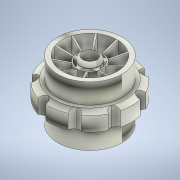
# Autodesk Inventor part: ozubene-kolo_mini
Saved by Autodesk Inventor 2022 (Build 260153000, 153)
## iProperties
Created: 2022-11-27
Part Number: ozubene-kolo_mini
Material: Generic
Document SubType Name: Modeling
Designer: matys
Density: 1 g/cm^3
Appearance: Running - Light Gray
Author: matys
Autodesk Inventor part; units mm, degrees
ref_plane "YZ Plane" through (0, 0, 0) normal (1, 0, 0) x (0, 1, 0)
ref_plane "XZ Plane" through (0, 0, 0) normal (0, 1, 0) x (-1, 0, 0)
ref_plane "XY Plane" through (0, 0, 0) normal (0, 0, 1) x (1, 0, 0)
sketch "Sketch1" plane through (0, 0, 0) normal (0, 1, 0) x (-1, 0, 0)
  line L0 (0, 0) -> (15, 0)
  circle A0 centre (0, 0) radius 15
  dimension "d0" = 15
  constraints: 2 end point, 1 coincident, 1 horizontal, 1 horizontal alignment, 2 other
  measures "d0" distance of L0.start L0.end
extrude "Extrusion1" add sketch "Sketch1" along normal blind 8.5
sketch "Sketch2" plane through (0, 8.5, 0) normal (0, 1, 0) x (1, 0, 0)
  line L0 (0, 0) -> (-15, 0)
  circle A0 centre (0, 0) radius 15 projected
  line L1 (-15, 0) -> (-19, 0)
  circle A1 centre (0, 0) radius 15
  line L2 (-15, 0) -> (-17.5, 0)
  circle A2 centre (0, 0) radius 17.5
  dimension "d10" = 2.5
  constraints: 6 end point, 2 coincident, 2 horizontal alignment, 2 point on line, 1 centre point, 1 horizontal, 4 other
  measures "d10" distance of L0.end L2.end
extrude "Extrusion2" add sketch "Sketch2" along normal blind 8 contours A0 | A2
sketch "Sketch3" plane through (0, 16.5, 0) normal (0, 1, 0) x (1, 0, 0)
  line L0 (0, 0) -> (-15, 0)
  circle A0 centre (0, 0) radius 15
  constraints: 2 end point, 1 coincident, 1 horizontal, 1 horizontal alignment, 2 other
extrude "Extrusion3" add sketch "Sketch3" along normal blind 8.5
sketch "Sketch5" plane through (0, 16.5, 0) normal (0, 1, 0) x (1, 0, 0)
  circle A0 centre (0, 0) radius 17.5 projected
  line L0 (0, 0) -> (-17.5, 0)
  line L1 (0, 2) -> (-17.3853, 2)
  line L2 (0, -2) -> (-17.3853, -2)
  circle A1 centre (0, 0) radius 15 projected
  circle A2 centre (0, 0) radius 17.5
  arc A3 (-17.3853, -2) -> (-15, 0) centre (-17.3426, 0.3715) ccw
  arc A4 (-15, 0) -> (-17.3853, 2) centre (-17.3426, -0.3715) ccw
  line L3 (-17.5, 0) -> (-13.1342, 11.5644)
  arc A5 (-11.4907, -9.6418) -> (-14.6035, -9.643) centre (-13.0464, -11.4322) ccw
  arc A6 (-12.0324, -12.7072) -> (-11.4907, -9.6418) centre (-13.524, -10.863) ccw
  arc A7 (-2.6047, -14.7721) -> (-4.9885, -16.7739) centre (-2.6456, -17.1437) ccw
  arc A8 (-1.0493, -17.4685) -> (-2.6047, -14.7721) centre (-3.3774, -17.0146) ccw
  arc A9 (7.5, -12.9904) -> (6.9606, -16.0561) centre (8.9931, -14.8334) ccw
  arc A10 (10.4247, -14.0561) -> (7.5, -12.9904) centre (8.3496, -15.2049) ccw
  arc A11 (14.0954, -5.1303) -> (15.6528, -7.8255) centre (16.4238, -5.5824) ccw
  arc A12 (17.0209, -4.0668) -> (14.0954, -5.1303) centre (16.1697, -6.2807) ccw
  arc A13 (14.0954, 5.1303) -> (17.0209, 4.0668) centre (16.1697, 6.2807) ccw
  arc A14 (15.6528, 7.8255) -> (14.0954, 5.1303) centre (16.4238, 5.5824) ccw
  arc A15 (7.5, 12.9904) -> (10.4247, 14.0561) centre (8.3496, 15.2049) ccw
  arc A16 (6.9606, 16.0561) -> (7.5, 12.9904) centre (8.9931, 14.8334) ccw
  arc A17 (-2.6047, 14.7721) -> (-1.0493, 17.4685) centre (-3.3774, 17.0146) ccw
  arc A18 (-4.9885, 16.7739) -> (-2.6047, 14.7721) centre (-2.6456, 17.1437) ccw
  arc A19 (-11.4907, 9.6418) -> (-12.0324, 12.7072) centre (-13.524, 10.863) ccw
  arc A20 (-14.6035, 9.643) -> (-11.4907, 9.6418) centre (-13.0464, 11.4322) ccw
  point P0 (-14.6035, -9.643)
  point P1 (-1.0493, -17.4685)
  point P2 (15.6528, -7.8255)
  point P3 (17.0209, 4.0668)
  point P4 (10.4247, 14.0561)
  point P5 (-1.0493, 17.4685)
  point P6 (-17.2999, -2)
  point P7 (-16.7712, 1.9305)
  point P8 (-17.2999, 2)
  dimension "d11" = 2
  dimension "d12" = 2
  dimension "d14" = 12.361
  dimension "d17" = 360
  constraints: 41 point on circle, 19 centre point, 8 end point, 2 parallel, 2 symmetric about line, 1 coincident, 1 horizontal, 1 horizontal alignment, 1 point on line, 66 other
  measures "d11" distance between parallel lines of L0 L1
  measures "d12" distance between parallel lines of L0 L2
  measures "d14" distance of L0.end L3.end
extrude "Extrusion4" cut sketch "Sketch5" against normal blind 8.5 contours A13 A14 A0 | A0 A11 A12 | A15 A16 A0 | A0 A9 A10 | A18 A0 A17 | A8 A0 A7 | A20 L3 A0 A19 | A0 L0 A3 | A6 A0 A5 | A20 A0 L3 | L0 L3 A4 | A4 L3 A0
chamfer "Chamfer1" distance 2.5 distance2 1 1 edges at (13.4058, 16.5, 11.2488) measured on face at (13.0228, 16.5, 10.9274)
chamfer "Chamfer2" distance 2.5 distance2 1 1 edges at (3.0388, 16.5, 17.2341) measured on face at (2.952, 16.5, 16.7417)
chamfer "Chamfer3" distance 2.5 distance2 1 1 edges at (-8.75, 16.5, 15.1554) measured on face at (-8.5, 16.5, 14.7224)
chamfer "Chamfer4" distance 2.5 distance2 1 1 edges at (-16.4446, 16.5, 5.9854) measured on face at (-15.9748, 16.5, 5.8143)
chamfer "Chamfer5" distance 2.5 distance2 1 1 edges at (-16.4446, 16.5, -5.9854) measured on face at (-15.9748, 16.5, -5.8143)
chamfer "Chamfer6" distance 2.5 distance2 1 1 edges at (-8.75, 16.5, -15.1554) measured on face at (-8.5, 16.5, -14.7224)
chamfer "Chamfer7" distance 2.5 distance2 1 1 edges at (3.0388, 16.5, -17.2341) measured on face at (2.952, 16.5, -16.7417)
chamfer "Chamfer8" distance 2.5 distance2 1 1 edges at (13.4058, 16.5, -11.2488) measured on face at (13.0228, 16.5, -10.9274)
chamfer "Chamfer9" distance 2.5 distance2 1 1 edges at (17.5, 16.5, 0) measured on face at (17, 16.5, 0)
chamfer "Chamfer10" distance 1 distance2 2.5 1 edges at (13.4058, 8.5, 11.2488) measured on face at (13.4058, 9, 11.2488)
chamfer "Chamfer11" distance 1 distance2 2.5 1 edges at (3.0388, 8.5, 17.2341) measured on face at (3.0388, 9, 17.2341)
chamfer "Chamfer12" distance 1 distance2 2.5 1 edges at (-8.75, 8.5, 15.1554) measured on face at (-8.75, 9, 15.1554)
chamfer "Chamfer13" distance 1 distance2 2.5 1 edges at (-16.4446, 8.5, 5.9854) measured on face at (-16.4446, 9, 5.9854)
chamfer "Chamfer14" distance 1 distance2 2.5 1 edges at (-16.4446, 8.5, -5.9854) measured on face at (-16.4446, 9, -5.9854)
chamfer "Chamfer15" distance 1 distance2 2.5 1 edges at (-8.75, 8.5, -15.1554) measured on face at (-8.75, 9, -15.1554)
chamfer "Chamfer16" distance 1 distance2 2.5 1 edges at (3.0388, 8.5, -17.2341) measured on face at (3.0388, 9, -17.2341)
chamfer "Chamfer17" distance 1 distance2 2.5 1 edges at (13.4058, 8.5, -11.2488) measured on face at (13.4058, 9, -11.2488)
chamfer "Chamfer18" distance 1 distance2 2.5 1 edges at (17.5, 8.5, 0) measured on face at (17.5, 9, 0)
sketch "Sketch6" plane through (0, 25, 0) normal (0, 1, 0) x (1, 0, 0)
  circle A0 centre (0, 0) radius 15
  circle A1 centre (0, 0) radius 15 projected
  line L0 (0, -15) -> (0, -13.5)
  circle A2 centre (0, 0) radius 13.5
  dimension "d75" = 1.5
  constraints: 2 coincident, 2 end point, 2 vertical alignment, 1 centre point, 1 vertical, 3 other
  measures "d75" distance of L0.start L0.end
extrude "Extrusion5" cut sketch "Sketch6" against normal blind 8.5
sketch "Sketch7" plane through (0, 0, 0) normal (0, -1, 0) x (1, 0, 0)
  circle A0 centre (0, 0) radius 15
  arc A1 (-2.6047, -14.7721) -> (7.5, -12.9904) centre (0, 0) ccw projected
  line L0 (0, -15) -> (0, -13.5)
  circle A2 centre (0, 0) radius 13.5
  dimension "d78" = 1.5
  constraints: 2 coincident, 2 end point, 1 centre point, 1 point on circle, 1 vertical, 1 vertical alignment, 2 other
  measures "d78" distance of L0.start L0.end
extrude "Extrusion6" cut sketch "Sketch7" against normal blind 8.5
sketch "Sketch8" plane through (0, 25, 0) normal (0, 1, 0) x (1, 0, 0)
  circle A0 centre (0, 0) radius 3
  dimension "d81" = 6
  constraints: 1 centre point, 1 coincident
  measures "d81" diameter of A0
extrude "Extrusion7" cut sketch "Sketch8" against normal blind 3.2
sketch "Sketch9" plane through (0, 21.8, 0) normal (0, 1, 0) x (1, 0, 0)
  circle A0 centre (0, 0) radius 2
  dimension "d84" = 4
  constraints: 1 centre point, 1 coincident
  measures "d84" diameter of A0
extrude "Extrusion8" cut sketch "Sketch9" against normal blind 5
sketch "Sketch10" plane through (0, 16.8, 0) normal (0, 1, 0) x (1, 0, 0)
  circle A0 centre (0, 0) radius 2 projected
  line L0 (2.2828, 0) -> (0, -2.2828)
  line L1 (0, -2.2828) -> (-2.2828, 0)
  line L2 (-2.2828, 0) -> (0, 2.2828)
  line L3 (0, 2.2828) -> (2.2828, 0)
  point P0 (1.9764, 0.3065)
  point P1 (0.3065, 1.9764)
  point P2 (-0.3065, 1.9764)
  point P3 (-1.9764, 0.3065)
  point P4 (-1.9764, -0.3065)
  point P5 (-0.3065, -1.9764)
  point P6 (0.3065, -1.9764)
  point P7 (1.9764, -0.3065)
  constraints: 8 end point, 2 parallel, 1 perpendicular
extrude "Extrusion9" cut sketch "Sketch10" against normal blind 6 contours A0 L0 L1 L2 L3
sketch "Sketch11" plane through (0, 10.8, 0) normal (0, 1, 0) x (1, 0, 0)
  circle A0 centre (0, 0) radius 1.15
  dimension "d90" = 2.3
  constraints: 1 centre point, 1 coincident
  measures "d90" diameter of A0
extrude "Extrusion10" cut sketch "Sketch11" against normal through all
sketch "Sketch12" plane through (0, 25, 0) normal (0, 1, 0) x (1, 0, 0)
  circle A0 centre (0, 0) radius 3 projected
  circle A1 centre (0, 0) radius 13.5 projected
  line L0 (0, -13.5) -> (0, -11.5)
  circle A2 centre (0, 0) radius 11.5
  circle A3 centre (0, 0) radius 2 projected
  line L1 (-0.35, -11.4947) -> (-0.35, -5.4889)
  line L2 (0, 0) -> (0, -5.5)
  circle A4 centre (0, 0) radius 5.5
  line L3 (0.35, -11.4947) -> (0.35, -5.4889)
  line L4 (6.4732, -9.5051) -> (2.9431, -4.6463)
  line L5 (7.0396, -9.0937) -> (3.5094, -4.2348)
  line L6 (10.8239, -3.8849) -> (5.1121, -2.029)
  line L7 (11.0402, -3.2192) -> (5.3284, -1.3633)
  line L8 (11.0402, 3.2192) -> (5.3284, 1.3633)
  line L9 (10.8239, 3.8849) -> (5.1121, 2.029)
  line L10 (7.0396, 9.0937) -> (3.5094, 4.2348)
  line L11 (6.4732, 9.5051) -> (2.9431, 4.6463)
  line L12 (0.35, 11.4947) -> (0.35, 5.4889)
  line L13 (-0.35, 11.4947) -> (-0.35, 5.4889)
  line L14 (-6.4732, 9.5051) -> (-2.9431, 4.6463)
  line L15 (-7.0396, 9.0937) -> (-3.5094, 4.2348)
  line L16 (-10.8239, 3.8849) -> (-5.1121, 2.029)
  line L17 (-11.0402, 3.2192) -> (-5.3284, 1.3633)
  line L18 (-11.0402, -3.2192) -> (-5.3284, -1.3633)
  line L19 (-10.8239, -3.8849) -> (-5.1121, -2.029)
  line L20 (-7.0396, -9.0937) -> (-3.5094, -4.2348)
  line L21 (-6.4732, -9.5051) -> (-2.9431, -4.6463)
  line L22 (0, -5.5) -> (0, -5)
  circle A5 centre (0, 0) radius 5
  circle A6 centre (0, 0) radius 1.15 projected
  line L23 (3.2642, -2.6284) -> (1.4936, -3.9149)
  line L24 (0.7458, -4.9441) -> (1.4936, -3.9149)
  line L25 (4.4718, -2.2367) -> (3.2642, -2.6284)
  line L26 (4.9326, -0.8185) -> (4.1848, 0.2107)
  line L27 (3.5085, 2.2922) -> (4.1848, 0.2107)
  line L28 (3.5091, 3.5618) -> (3.5085, 2.2922)
  line L29 (2.3027, 4.4382) -> (1.0928, 4.0451)
  line L30 (-1.0959, 4.0451) -> (1.0928, 4.0451)
  line L31 (-2.3031, 4.438) -> (-1.0959, 4.0451)
  line L32 (-3.5094, 3.5615) -> (-3.5094, 2.2893)
  line L33 (-4.1857, 0.2078) -> (-3.5094, 2.2893)
  line L34 (-4.9325, -0.819) -> (-4.1857, 0.2078)
  line L35 (-4.4716, -2.2371) -> (-3.2617, -2.6302)
  line L36 (-1.4911, -3.9167) -> (-3.2617, -2.6302)
  line L37 (-0.7454, -4.9441) -> (-1.4911, -3.9167)
  dimension "d93" = 2
  dimension "d96" = 5.5
  dimension "d99" = 360
  dimension "d101" = 0.5
  dimension "d104" = 360
  constraints: 76 end point, 9 point on circle, 5 coincident, 3 centre point, 1 point on line, 1 vertical alignment, 98 other
  measures "d93" distance of L0.start L0.end
  measures "d96" distance of L2.start L2.end
  measures "d101" distance of L2.end L22.end
extrude "Extrusion11" cut sketch "Sketch12" against normal through all contours A2 L7 A4 L8 | L9 A4 L10 A2 | A2 L5 A4 L6 | L11 A4 L12 A2 | A2 L3 A4 L4 | L13 A4 L14 A2 | A2 L21 A4 L1 | L15 A4 L16 A2 | A2 L19 A4 L20 | L17 A4 L18 A2 | A5 L26 L27 L28 | L29 L30 L31 A5 | A5 L24 L23 L25 | L32 L33 L34 A5 | A5 L35 L36 L37
sketch "Sketch13" plane through (0, 25, 0) normal (0, 1, 0) x (1, 0, 0)
  circle A0 centre (0, 0) radius 5.5
  circle A1 centre (0, 0) radius 1.15 projected
  circle A2 centre (0, 0) radius 4.0451
  point P0 (-5.1121, -2.029)
  constraints: 2 coincident, 1 centre point, 3 other
extrude "Extrusion12" cut sketch "Sketch13" against normal blind 2 contours A0
fillet "Fillet2" radius 2 6 edges at (3.9953, 25, -0.6328) (2.3776, 25, -3.2725) (-2.3776, 25, -3.2725) (-3.8471, 25, 1.25) (0, 25, 4.0451) (3.6042, 25, 1.8364)
chamfer "Chamfer20" distance 6 distance2 2 1 edges at (3.2328, 25, 4.4496) measured on face at (3.5267, 25, 4.8541)
chamfer "Chamfer21" distance 6 distance2 2 1 edges at (0, 25, 5.5) measured on face at (0, 25, 6)
chamfer "Chamfer22" distance 6 distance2 2 1 edges at (-3.2328, 25, 4.4496) measured on face at (-3.5267, 25, 4.8541)
chamfer "Chamfer23" distance 6 distance2 2 1 edges at (-5.2308, 25, 1.6996) measured on face at (-5.7063, 25, 1.8541)
chamfer "Chamfer24" distance 6 distance2 2 1 edges at (-5.2308, 25, -1.6996) measured on face at (-5.7063, 25, -1.8541)
chamfer "Chamfer25" distance 6 distance2 2 1 edges at (-3.2328, 25, -4.4496) measured on face at (-3.5267, 25, -4.8541)
chamfer "Chamfer26" distance 6 distance2 2 1 edges at (0, 25, -5.5) measured on face at (0, 25, -6)
chamfer "Chamfer27" distance 6 distance2 2 1 edges at (3.2328, 25, -4.4496) measured on face at (3.5267, 25, -4.8541)
chamfer "Chamfer28" distance 6 distance2 2 1 edges at (5.2308, 25, -1.6996) measured on face at (5.7063, 25, -1.8541)
chamfer "Chamfer29" distance 6 distance2 2 1 edges at (5.2308, 25, 1.6996) measured on face at (5.7063, 25, 1.8541)
body "Solid1"
